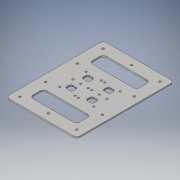
# Autodesk Inventor part: Telapak
Saved by Autodesk Inventor 2016 (Build 200138000, 138)
## iProperties
Created: 2017-02-04
Part Number: Telapak
Material: Generic
Document SubType Name: Modeling
Designer: Ghana
Density: 1 g/cm^3
Appearance: Default
Author: Ghana
Autodesk Inventor part; units mm, degrees
ref_plane "YZ Plane" through (0, 0, 0) normal (1, 0, 0) x (0, 1, 0)
ref_plane "XZ Plane" through (0, 0, 0) normal (0, 1, 0) x (-1, 0, 0)
ref_plane "XY Plane" through (0, 0, 0) normal (0, 0, 1) x (1, 0, 0)
sketch "Sketch1" plane through (0, 0, 0) normal (0, 1, 0) x (-1, 0, 0)
  circle A0 centre (97, -135) radius 1.5
  circle A1 centre (97, -15) radius 1.5
  circle A2 centre (15, -135) radius 1.5
  circle A3 centre (15, -15) radius 1.5
  circle A4 centre (56, -135) radius 1.5
  circle A5 centre (56, -15) radius 1.5
  circle A6 centre (97, -97.9289) radius 1.5
  circle A7 centre (97, -52.0711) radius 1.5
  circle A8 centre (15, -97.9289) radius 1.5
  circle A9 centre (15, -52.0711) radius 1.5
  circle A10 centre (31.5, -94) radius 1.3
  circle A11 centre (53.5, -94) radius 1.3
  circle A12 centre (53.5, -56) radius 1.3
  circle A13 centre (31.5, -56) radius 1.3
  circle A14 centre (53.5, -75) radius 1.3
  circle A15 centre (31.5, -75) radius 1.3
  line L0 (84.9289, -42.0711) -> (27.0711, -42.0711)
  line L1 (22.0711, -37.0711) -> (22.0711, -27.0711)
  line L2 (27.0711, -22.0711) -> (84.9289, -22.0711)
  line L3 (89.9289, -27.0711) -> (89.9289, -37.0711)
  line L4 (27.0711, -127.9289) -> (84.9289, -127.9289)
  line L5 (89.9289, -122.9289) -> (89.9289, -112.9289)
  line L6 (84.9289, -107.9289) -> (27.0711, -107.9289)
  line L7 (22.0711, -112.9289) -> (22.0711, -122.9289)
  line L8 (39, -91.5) -> (43, -91.5)
  line L9 (46, -88.5) -> (46, -85.5)
  line L10 (43, -82.5) -> (39, -82.5)
  line L11 (36, -85.5) -> (36, -88.5)
  line L12 (43, -58.5) -> (39, -58.5)
  line L13 (36, -61.5) -> (36, -64.5)
  line L14 (39, -67.5) -> (43, -67.5)
  line L15 (46, -64.5) -> (46, -61.5)
  arc A16 (84.9289, -127.9289) -> (89.9289, -122.9289) centre (84.9289, -122.9289) ccw
  arc A17 (22.0711, -122.9289) -> (27.0711, -127.9289) centre (27.0711, -122.9289) ccw
  arc A18 (27.0711, -107.9289) -> (22.0711, -112.9289) centre (27.0711, -112.9289) ccw
  arc A19 (89.9289, -112.9289) -> (84.9289, -107.9289) centre (84.9289, -112.9289) ccw
  arc A20 (84.9289, -42.0711) -> (89.9289, -37.0711) centre (84.9289, -37.0711) ccw
  arc A21 (89.9289, -27.0711) -> (84.9289, -22.0711) centre (84.9289, -27.0711) ccw
  arc A22 (27.0711, -22.0711) -> (22.0711, -27.0711) centre (27.0711, -27.0711) ccw
  arc A23 (22.0711, -37.0711) -> (27.0711, -42.0711) centre (27.0711, -37.0711) ccw
  arc A24 (43, -91.5) -> (46, -88.5) centre (43, -88.5) ccw
  arc A25 (36, -88.5) -> (39, -91.5) centre (39, -88.5) ccw
  arc A26 (39, -82.5) -> (36, -85.5) centre (39, -85.5) ccw
  arc A27 (46, -85.5) -> (43, -82.5) centre (43, -85.5) ccw
  arc A28 (43, -67.5) -> (46, -64.5) centre (43, -64.5) ccw
  arc A29 (36, -64.5) -> (39, -67.5) centre (39, -64.5) ccw
  arc A30 (39, -58.5) -> (36, -61.5) centre (39, -61.5) ccw
  arc A31 (46, -61.5) -> (43, -58.5) centre (43, -61.5) ccw
  circle A32 centre (42.5, -75) radius 1.3
  circle A33 centre (80.5, -94) radius 1.3
  circle A34 centre (58.5, -94) radius 1.3
  circle A35 centre (58.5, -56) radius 1.3
  circle A36 centre (80.5, -56) radius 1.3
  circle A37 centre (58.5, -75) radius 1.3
  circle A38 centre (80.5, -75) radius 1.3
  line L16 (73, -91.5) -> (69, -91.5)
  line L17 (66, -88.5) -> (66, -85.5)
  line L18 (69, -82.5) -> (73, -82.5)
  line L19 (76, -85.5) -> (76, -88.5)
  line L20 (69, -58.5) -> (73, -58.5)
  line L21 (76, -61.5) -> (76, -64.5)
  line L22 (73, -67.5) -> (69, -67.5)
  line L23 (66, -64.5) -> (66, -61.5)
  arc A39 (66, -88.5) -> (69, -91.5) centre (69, -88.5) ccw
  arc A40 (73, -91.5) -> (76, -88.5) centre (73, -88.5) ccw
  arc A41 (76, -85.5) -> (73, -82.5) centre (73, -85.5) ccw
  arc A42 (69, -82.5) -> (66, -85.5) centre (69, -85.5) ccw
  arc A43 (66, -64.5) -> (69, -67.5) centre (69, -64.5) ccw
  arc A44 (73, -67.5) -> (76, -64.5) centre (73, -64.5) ccw
  arc A45 (76, -61.5) -> (73, -58.5) centre (73, -61.5) ccw
  arc A46 (69, -58.5) -> (66, -61.5) centre (69, -61.5) ccw
  circle A47 centre (69.5, -75) radius 1.3
  line L24 (10, -5) -> (102, -5)
  line L25 (107, -10) -> (107, -140)
  line L26 (102, -145) -> (10, -145)
  line L27 (5, -140) -> (5, -10)
  arc A48 (102, -145) -> (107, -140) centre (102, -140) ccw
  arc A49 (5, -140) -> (10, -145) centre (10, -140) ccw
  arc A50 (10, -5) -> (5, -10) centre (10, -10) ccw
  arc A51 (107, -10) -> (102, -5) centre (102, -10) ccw
  dimension "d24" = 3
  dimension "d25" = 3
  dimension "d26" = 3
  dimension "d27" = 3
  dimension "d28" = 3
  dimension "d29" = 3
  dimension "d30" = 3
  dimension "d32" = 3
  dimension "d47" = 5
  dimension "d48" = 5
  dimension "d59" = 5
  dimension "d60" = 10
  dimension "d61" = 10
  dimension "d67" = 2.6
  dimension "d71" = 140
  dimension "d72" = 102
  constraints: 56 end point, 56 point on circle, 52 centre point, 40 tangent, 23 equal radius, 10 parallel, 6 vertical alignment, 5 perpendicular, 3 horizontal alignment, 1 horizontal
  measures "d24" diameter of A0
  measures "d25" diameter of A2
  measures "d26" diameter of A6
  measures "d27" diameter of A8
  measures "d28" diameter of A7
  measures "d29" diameter of A1
  measures "d30" diameter of A5
  measures "d32" diameter of A9
  measures "d47" radius of A16
  measures "d48" radius of A20
  measures "d59" radius of A48
  measures "d60" distance from line of L25 A0.centre
  measures "d61" distance from line of A0.centre L26
  measures "d67" diameter of A10
  measures "d71" distance between parallel lines of L24 L26
  measures "d72" distance between parallel lines of L27 L25
extrude "Extrusion2" add sketch "Sketch1" along normal blind 2
body "Solid2"
